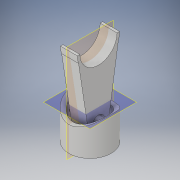
# Autodesk Inventor part: PistonTest2
Saved by Autodesk Inventor 2018 (Build 220112000, 112)
## iProperties
Created: 2019-08-30
Part Number: PistonTest2
Material: Generic
Document SubType Name: Modeling
Designer: 871357
Density: 1 g/cm^3
Appearance: Default
Author: 871357
Autodesk Inventor part; units mm, degrees
ref_plane "XZ Plane" through (0, 0, 0) normal (0, 1, 0) x (-1, 0, 0)
ref_plane "XY Plane" through (0, 0, 0) normal (0, 0, 1) x (1, 0, 0)
sketch "Sketch1" plane through (0, 0, 0) normal (0, 1, 0) x (-1, 0, 0)
  circle A0 centre (0, 0) radius 6.35
  dimension "d0" = 12.7
  constraints: 1 centre point, 1 coincident
  measures "d0" diameter of A0
extrude "Extrusion1" add sketch "Sketch1" along normal blind 7.62
sketch "Sketch2" plane through (0, 0, 0) normal (0, 0, 1) x (1, 0, 0)
  line L0 (6.35, 7.62) -> (-6.35, 7.62) projected
  arc A0 (-6.35, 7.62) -> (6.35, 7.62) centre (0, 13.97) ccw
  line L1 (-6.35, 7.62) -> (-6.35, 5.08) construction
  line L2 (-6.35, 0) -> (-6.35, 7.62) construction
  point P0 (0, 0)
  dimension "d5" = 2.54
  dimension "d6" = 8.89
  constraints: 2 end point, 2 point on circle, 1 centre point, 1 point on line
  measures "d5" distance of L0.end L1.end
  measures "d6" vertical distance of L1.end A0.centre
extrude "Extrusion2" cut sketch "Sketch2" along normal mid plane 25.4
ref_plane "Work Plane1" through (0, 7.62, 0) normal (0, -1, 0) x (1, 0, 0)
sketch "Sketch3" plane through (0, 7.62, 0) normal (0, -1, 0) x (1, 0, 0)
  circle A0 centre (0, 0) radius 5.08
  dimension "d10" = 10.16
  constraints: 1 centre point, 1 coincident
  measures "d10" diameter of A0
extrude "Extrusion3" cut sketch "Sketch3" along normal blind 6.35
sketch "Sketch4" plane through (0, 0, 0) normal (1, 0, 0) x (0, 1, 0)
  circle A0 centre (3.81, 0) radius 1.27
  line L0 (1.27, 5.08) -> (1.27, -5.08) projected
  point P0 (0, 0)
  dimension "d13" = 2.54
  dimension "d14" = 2.54
  constraints: 1 centre point
  measures "d13" diameter of A0
  measures "d14" distance from line of L0 A0.centre
extrude "Extrusion4" add sketch "Sketch4" along normal mid plane 11.43
sketch "Sketch6" plane through (0, 1.27, 0) normal (0, 1, 0) x (1, 0, 0)
  circle A0 centre (0, 0) radius 5.08 projected
extrude "Extrusion6" cut sketch "Sketch6" against normal blind 25.4
sketch "Sketch5" plane through (0, 0, 0) normal (1, 0, 0) x (0, 1, 0)
  circle A0 centre (3.81, 0) radius 1.778
  arc A1 (3.81, 3.175) -> (3.81, -3.175) centre (3.81, 0) ccw
  arc A2 (24.13, 5.588) -> (24.13, -5.588) centre (24.13, 0) ccw
  line L0 (24.13, 6.35) -> (24.13, 5.588)
  line L1 (24.13, -5.588) -> (24.13, -6.35)
  arc A3 (24.13, 6.35) -> (21.9635, 5.969) centre (24.13, 0) ccw
  arc A4 (21.9635, -5.969) -> (24.13, -6.35) centre (24.13, 0) ccw
  line L2 (3.81, 3.175) -> (21.9635, 5.969)
  line L3 (3.81, -3.175) -> (21.9635, -5.969)
  point P0 (0, 0)
  point P1 (3.81, 1.27)
  dimension "d17" = 3.556
  dimension "d18" = 6.35
  dimension "d21" = 11.176
  dimension "d22" = 0
  dimension "d23" = 20.32
  constraints: 8 end point, 8 point on circle, 5 centre point, 2 coincident, 2 vertical, 1 other
  measures "d17" diameter of A0
  measures "d18" diameter of A1
  measures "d21" diameter of A2
  measures "d22" vertical distance of A0.centre A2.centre
  measures "d23" distance of A2.centre A0.centre
extrude "Extrusion5" add sketch "Sketch5" along normal mid plane 5.08
sketch "Sketch7" plane through (0, 0, 0) normal (0, -1, 0) x (1, 0, 0)
  circle A0 centre (0, 0) radius 5.08 construction
  circle A1 centre (0, 0) radius 6.35 projected
extrude "Extrusion7" add sketch "Sketch7" along normal blind 2.54
sketch "Sketch8" plane through (0, 0, 0) normal (1, 0, 0) x (0, 1, 0)
  point P0 (0, 0)
body "Solid1"
